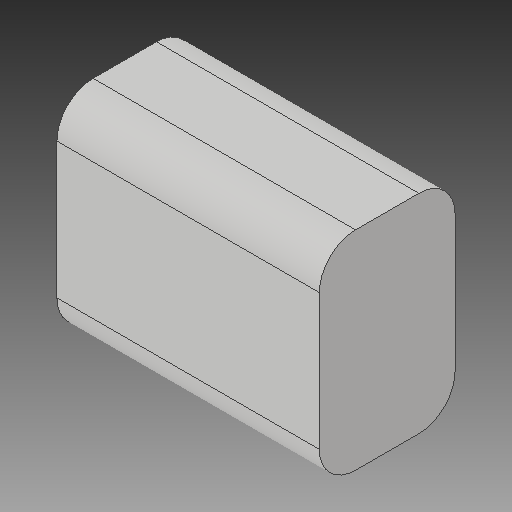
# Autodesk Inventor part: ＳＮ型電池ホルダー_SN3-6B
Saved by Autodesk Inventor 2017 (Build 210142000, 142)
## iProperties
Created: 2016-08-20
Part Number: ＳＮ型電池ホルダー_SN3-6B
Material: 一般
Document SubType Name: Modeling
Designer: NN
Density: 2.18597 g/cm^3
Appearance: 既定
Mass: 168 g
Surface Area: 106.695 cm^2
Volume: 76.8536 cm^3
Author: NN
Autodesk Inventor part; units mm, degrees
ref_plane "YZ Plane" through (0, 0, 0) normal (1, 0, 0) x (0, 1, 0)
ref_plane "XZ Plane" through (0, 0, 0) normal (0, 1, 0) x (-1, 0, 0)
ref_plane "XY Plane" through (0, 0, 0) normal (0, 0, 1) x (1, 0, 0)
sketch "スケッチ1" plane through (0, 0, 0) normal (0, 0, 1) x (1, 0, 0)
  line L0 (0, 0) -> (58, 0)
  line L1 (58, 0) -> (58, 46)
  line L2 (58, 46) -> (0, 46)
  line L3 (0, 46) -> (0, 0)
  dimension "d0" = 46
  dimension "d1" = 58
  constraints: 8 end point, 2 parallel, 1 horizontal, 1 perpendicular
  measures "d0" distance of L2.end L0.start
  measures "d1" distance of L0.start L0.end
extrude "押し出し1" add sketch "スケッチ1" along normal blind 30
fillet "フィレット1" radius 8 4 edges at (29, 0, 30) (29, 46, 30) (29, 0, 0) (29, 46, 0)
